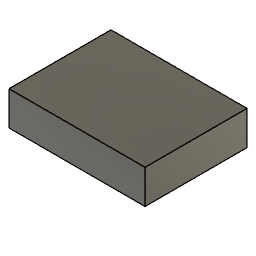
Cutting Block Tibia Shell (L&R) (Autodesk Fusion 360 design; units mm, degrees)
Autodesk Fusion 360 part; units mm, degrees
note: some values were not read from the file. Chosen so that the rebuilt part matches the saved one: which bodies a step acts on; which face or edge a step refers to. Set by a fixed rule: which sketch regions a step uses.
sketch "Sketch1" plane through (0, 0, 0) normal (0, 0, 1) x (1, 0, 0)
  line L0 (0, 64.6235) -> (0, -66.6531) construction
  line L1 (95.8471, 0) -> (-100, 0) construction
  circle A0 centre (18, 0) radius 20
  circle A1 centre (-18, 0) radius 20
  line L2 (40, 22) -> (-40, 22) construction
  line L3 (-40, 22) -> (-40, -22) construction
  line L4 (-40, -22) -> (40, -22) construction
  line L5 (40, -22) -> (40, 22) construction
  line L6 (40, 22) -> (-40, -22) construction
  line L7 (-40, 22) -> (40, -22) construction
  circle A2 centre (0, 80) radius 102
  line L8 (-18, 20) -> (18, 20)
  line L9 (-8.7733, 50.0836) -> (-8.7733, 13.6847)
  arc A3 (-8.7733, 13.6847) -> (8.7733, 13.6847) centre (0, 13.6847) ccw
  line L10 (8.7733, 13.6847) -> (8.7733, 50.0836)
  arc A4 (8.7733, 50.0836) -> (-8.7733, 50.0836) centre (0, 50.0836) ccw
  line L11 (0, 50.0836) -> (0, 13.6847) construction
  point P0 (0, 31.8841)
  dimension "d1" = 18
  dimension "d2" = 80
  dimension "d3" = 44
  dimension "d4" = 40
  constraint vertical L0
  constraint perpendicular L0 L1
  constraint coincident origin L0
  constraint coincident origin L1
  constraint coincident L1 A0.centre
  constraint coincident L1 A1.centre
  constraint equal A0 A1
  constraint horizontal L2
  constraint perpendicular L2 L3
  constraint parallel L2 L4
  constraint parallel L3 L5
  constraint coincident L6 origin
  constraint coincident L7 origin
  constraint symmetric L0 A0 A1
  constraint coincident L0 A2.centre
  constraint tangent A0 A2
  constraint tangent L4 A2
  constraint parallel L2 L8
  constraint tangent A1 L8
  constraint coincident A1 L8.start
  constraint coincident A0 L8.end
  constraint tangent L9 A3
  constraint tangent A3 L10
  constraint parallel L9 L10
  constraint tangent L10 A4
  constraint tangent L9 A4
  constraint coincident L0 A3.centre
  constraint perpendicular L8 L11
  constraint coincident L0 P0
  constraint midpoint L11 P0
  measures "d1" distance of L0 A0.centre
  measures "d2" distance of L2.start L2.end
  measures "d3" distance of L2.start L4.end
  measures "d4" diameter of A0
extrude "Extrude1" add sketch "Sketch1" along normal blind 5 contours A0 A1 A3 L10 | A0 L8 L10 | A0 A1 A2 | A0 A1 L9 A3 | A0 A1 A3 | A1 L8 L9 picked at (9.3284, -4.7386) picked at (-9.2755, -5.111) picked at (-0.6455, 1.124) makes body 1
fillet "Fillet2" radius 8 2 edges at (8.7733, 20, 2.5) (-8.7733, 20, 2.5) on bodies 1
extrude "Extrude3" add 1 faces at (0, -12.8446, 5) along direction (0, 0, 1) blind 5 separate body on bodies 1 makes body 2
shell "Shell2" thickness 2 removed faces 1 at (3.2154, -12.8497, 10) on bodies 2
sketch "Sketch4" plane through (0, 0, 0) normal (0, 0, -1) x (1, 0, 0)
  arc A0 (-16.6885, -20) -> (-8.729, -12.8035) centre (-16.6885, -12) ccw
  arc A1 (8.729, -12.8035) -> (-8.729, -12.8035) centre (0, -13.6847) ccw
  arc A2 (8.729, -12.8035) -> (16.6885, -20) centre (16.6885, -12) ccw
  line L0 (16.6885, -20) -> (18, -20)
  arc A3 (18, -20) -> (22.3902, 19.5122) centre (18, 0) ccw
  arc A4 (22.3902, 19.5122) -> (-22.3902, 19.5122) centre (0, -80) ccw
  arc A5 (-22.3902, 19.5122) -> (-18, -20) centre (-18, 0) ccw
  line L1 (-18, -20) -> (-16.6885, -20)
  circle A6 centre (0, 7) radius 3.5
  line L2 (0, 7) -> (14.0954, 1.8697) construction
  line L3 (-0.342, 6.0603) -> (13.7534, 0.93)
  arc A7 (13.7534, 0.93) -> (14.4374, 2.8094) centre (14.0954, 1.8697) ccw
  line L4 (14.4374, 2.8094) -> (0.342, 7.9397)
  arc A8 (0.342, 7.9397) -> (-0.342, 6.0603) centre (0, 7) ccw
  line L5 (0, 7) -> (14.0954, 1.8697) construction
  line L6 (0, -4.9114) -> (0, 22) construction
  line L7 (0, 7) -> (-14.0954, 1.8697) construction
  arc A9 (-14.4374, 2.8094) -> (-13.7534, 0.93) centre (-14.0954, 1.8697) ccw
  line L8 (0, 7) -> (-14.0954, 1.8697) construction
  arc A10 (0.342, 6.0603) -> (-0.342, 7.9397) centre (0, 7) ccw
  line L9 (-14.4374, 2.8094) -> (-0.342, 7.9397)
  line L10 (0.342, 6.0603) -> (-13.7534, 0.93)
  circle A11 centre (22, 10) radius 2.9
  circle A12 centre (22, -10) radius 2.9
  circle A13 centre (-22, 10) radius 2.9
  circle A14 centre (-22, -10) radius 2.9
  point P0 (0, 7)
  point P1 (-22.3902, 19.5122)
  point P2 (-18, 0)
  dimension "d18" = 7
  dimension "d19" = 7
  dimension "d20" = 2
  dimension "d21" = 70
  dimension "d22" = 15
  dimension "d32" = 5.8
  dimension "d33" = 22
  dimension "d34" = 20
  dimension "d35" = 10
  constraint vertical origin A6.centre
  constraint coincident P0 A6.centre
  constraint tangent L3 A7
  constraint tangent A7 L4
  constraint parallel L3 L4
  constraint tangent L4 A8
  constraint tangent L3 A8
  constraint coincident L2.end A7.centre
  constraint parallel L2 L5
  constraint midpoint A1 L6.start
  constraint midpoint A4 L6.end
  constraint symmetric P0 L6 A6.centre
  constraint symmetric L2.end L6 L7.end
  constraint symmetric L3.start L6 A10.start
  constraint symmetric L3.end L6 A9.end
  constraint symmetric A7.end L6 A9.start
  constraint symmetric L4.end L6 A10.end
  constraint symmetric A7 L6 A9
  constraint symmetric A8 L6 A10
  constraint equal A11 A12
  constraint vertical A11.centre A12.centre
  constraint symmetric A3.end L6 P1
  constraint symmetric A3.centre L6 P2
  constraint symmetric L6 A11 A13
  constraint symmetric L6 A12 A14
  measures "d18" diameter of A6
  measures "d19" distance of origin A6.centre
  measures "d20" distance of L3 L4
  measures "d21" angle of L2 L6
  measures "d22" distance of P0 L2.end
  measures "d32" diameter of A11
  measures "d33" distance of L6 A11.centre
  measures "d34" distance of A11.centre A12.centre
  measures "d35" vertical distance of origin A11.centre
extrude "Extrude4" add sketch "Sketch4" along normal blind 20 contours A6 L4 A8 A10 L9 | A6 L3 A8 L9 L10 | A6 A9 L9 L10 | A6 L3 A7 L4 | A6 L3 L4 A10 L10 | A6 L3 L10 bodies 1
sketch "Sketch5" plane through (0, 0, 0) normal (0, 1, 0) x (1, 0, 0)
  line L0 (0, -10) -> (0, 20) construction
  line L1 (-22.3902, -10) -> (22.3902, -10)
  line L2 (3.5, 20) -> (-3.5, 20)
  line L3 (0, 20) -> (16.4374, 20)
  line L4 (16.4374, 20) -> (16.4374, 0)
  line L5 (-22.3902, 0) -> (22.3902, 0)
  line L6 (14.4374, 0) -> (14.4374, 20)
  spline S0 degree 5 poles (0, 20) (0.3411, 19.8623) (1.0253, 19.654) (2.0582, 19.543) (3.4353, 19.7283) (5.0876, 20.1351) (6.592, 20.2718) (7.8837, 19.7528) (8.9451, 18.4166) (9.8035, 16.3217) (10.5137, 13.6618) (11.1462, 10.7153) (11.7741, 7.7829) (12.4628, 5.138) (13.2548, 2.959) (14.1714, 1.3345) (15.0111, 0.5059) (15.701, 0.1503) (16.1875, 0.0306) (16.4374, 0) knots 0 0 0 0 0 0 0.066667 0.133333 0.2 0.266667 0.333333 0.4 0.466667 0.533333 0.6 0.666667 0.733333 0.8 0.866667 0.933333 1 1 1 1 1 1
  line L7 (-3.7175, 21.5008) -> (3.7175, 18.4992)
  point P0 (7, 20)
  point P1 (12, 7)
  dimension "d25" = 2
  constraint vertical L0
  constraint coincident L0.start L1
  constraint coincident L0.end L2
  constraint coincident origin L0
  constraint perpendicular L0 L3
  constraint perpendicular L2 L4
  constraint coincident L4.end L5
  constraint midpoint L0.end L7
  measures "d25" distance of L4 L6
extrude "Extrude5" [suppressed]
mirror "Mirror1" [suppressed]
fillet "Fillet3" [suppressed]
extrude "Extrude6" add sketch "Sketch4" along normal blind 9 separate body contours A11 | A12 | A13 | A14 makes body 3 at (-19.1036, 10.1446, -6) makes body 4 at (24.8964, -9.8554, -6) makes body 5 at (-19.1036, -9.8554, -6) makes body 6 at (24.8964, 10.1446, -6)
chamfer "Chamfer1" distance 2.5 angle 45 4 edges at (-24.7037, 11.0487, -9) (19.2963, -8.9513, -9) (-24.7037, -8.9513, -9) (19.2963, 11.0487, -9) on bodies 3 4 5 6
combine "Combine1" operation add target body 1 tool bodies 6 4 2 3 5
move_face "OffsetFaces1" offset -1 1 faces at (0, -12.2976, 7) on bodies 1
sketch "Sketch6" plane through (0, 0, 10) normal (0, 0, 1) x (-1, 0, 0)
  arc A0 (10.7189, -12.6026) -> (16.6885, -18) centre (16.6885, -12) ccw
  arc A1 (10.7189, -12.6026) -> (-10.7189, -12.6026) centre (0, -13.6847) ccw
  arc A2 (-16.6885, -18) -> (-10.7189, -12.6026) centre (-16.6885, -12) ccw
  line L0 (-16.6885, -18) -> (-18, -18)
  arc A3 (-21.9512, 17.561) -> (-18, -18) centre (-18, 0) ccw
  arc A4 (21.9512, 17.561) -> (-21.9512, 17.561) centre (0, -80) ccw
  arc A5 (18, -18) -> (21.9512, 17.561) centre (18, 0) ccw
  line L1 (18, -18) -> (16.6885, -18)
  arc A6 (8.729, -12.8035) -> (16.6885, -20) centre (16.6885, -12) ccw
  line L2 (16.6885, -20) -> (18, -20)
  arc A7 (18, -20) -> (22.3902, 19.5122) centre (18, 0) ccw
  arc A8 (22.3902, 19.5122) -> (-22.3902, 19.5122) centre (0, -80) ccw
  arc A9 (-22.3902, 19.5122) -> (-18, -20) centre (-18, 0) ccw
  line L3 (-18, -20) -> (-16.6885, -20)
  arc A10 (-16.6885, -20) -> (-8.729, -12.8035) centre (-16.6885, -12) ccw
  arc A11 (8.729, -12.8035) -> (-8.729, -12.8035) centre (0, -13.6847) ccw
  line L4 (0, -4.9114) -> (0, 22)
  line L5 (1, -3.9114) -> (-1, -3.9114)
  line L6 (-1, -3.9114) -> (-1, 21)
  line L7 (-1, 21) -> (1, 21)
  line L8 (1, 21) -> (1, -3.9114)
  line L9 (2, -3.9114) -> (-2, -3.9114)
  line L10 (-2, -3.9114) -> (-2, 21)
  line L11 (-2, 21) -> (2, 21)
  line L12 (2, 21) -> (2, -3.9114)
  dimension "d40" = 2
  dimension "d41" = 1
  dimension "d42" = 1
  dimension "d44" = 2
  dimension "d45" = 1
  dimension "d46" = 1
  constraint midpoint A11 L4.start
  constraint midpoint A8 L4.end
  constraint horizontal L5
  constraint vertical L6
  constraint horizontal L7
  constraint vertical L8
  constraint horizontal L9
  constraint vertical L10
  constraint horizontal L11
  constraint vertical L12
  constraint collinear L5 L9
  constraint collinear L7 L11
  measures "d40" distance of L6 L8
  measures "d41" distance of L4.end L7
  measures "d42" distance of L4.start L5
  measures "d45" distance of L8 L12
  measures "d46" distance of L6 L10
extrude "Extrude7" add sketch "Sketch6" against normal up to surface (4 mm away) contours A1 A4 L4 L8 | A1 A4 L4 L6 bodies 1
extrude "Extrude8" add sketch "Sketch6" against normal blind 1 contours A1 A4 L8 L12 | A1 A4 L6 L10 bodies 1
chamfer "Chamfer3" distance 1 distance2 6.5 4 edges at (19.2963, -8.9513, -6.5) (19.2963, 11.0487, -6.5) (-24.7037, 11.0487, -6.5) (-24.7037, -8.9513, -6.5) measured on face at (21.1435, -7.8176, -7.0556) measured on face at (21.1435, 12.1824, -7.0556) measured on face at (-22.8565, 12.1824, -7.0556) measured on face at (-22.8565, -7.8176, -7.0556) on bodies 1
move_face "OffsetFaces2" offset -0.2 8 faces at (10.7896, -4.1371, -6.6667) (3.4994, -7.0641, -13.3333) (-10.7896, -4.1371, -6.6667) (-6.4577, -3.5854, -6.6667) (-1.0699, -3.6675, -13.3333) (6.4577, -3.5854, -13.3333) (14.3865, -0.913, -13.3333) (-13.9085, -0.8873, -13.3333) on bodies 1
sketch "Sketch7" plane through (0, 0, 0) normal (0, 0, -1) x (1, 0, 0)
  arc A0 (-16.6885, -20) -> (-8.729, -12.8035) centre (-16.6885, -12) ccw
  arc A1 (8.729, -12.8035) -> (-8.729, -12.8035) centre (0, -13.6847) ccw
  arc A2 (8.729, -12.8035) -> (16.6885, -20) centre (16.6885, -12) ccw
  line L0 (16.6885, -20) -> (18, -20)
  arc A3 (18, -20) -> (22.3902, 19.5122) centre (18, 0) ccw
  arc A4 (22.3902, 19.5122) -> (-22.3902, 19.5122) centre (0, -80) ccw
  arc A5 (-22.3902, 19.5122) -> (-18, -20) centre (-18, 0) ccw
  line L1 (-18, -20) -> (-16.6885, -20)
  line L2 (-14.369, 2.6215) -> (-3.2821, 6.6568)
  arc A6 (3.2821, 6.6568) -> (-3.2821, 6.6568) centre (0, 7) ccw
  line L3 (3.2821, 6.6568) -> (14.369, 2.6215)
  arc A7 (13.8218, 1.1179) -> (14.369, 2.6215) centre (14.0954, 1.8697) ccw
  line L4 (13.8218, 1.1179) -> (2.7349, 5.1532)
  arc A8 (-2.7349, 5.1532) -> (2.7349, 5.1532) centre (0, 7) ccw
  line L5 (-2.7349, 5.1532) -> (-13.8218, 1.1179)
  arc A9 (-14.369, 2.6215) -> (-13.8218, 1.1179) centre (-14.0954, 1.8697) ccw
  line L6 (80, 60) -> (-80, 60)
  line L7 (-80, 60) -> (-80, -60)
  line L8 (-80, -60) -> (80, -60)
  line L9 (80, -60) -> (80, 60)
  line L10 (80, 60) -> (-80, -60) construction
  line L11 (-80, 60) -> (80, -60) construction
  circle A10 centre (-22, 10) radius 2.9
  circle A11 centre (-22, -10) radius 2.9
  circle A12 centre (22, 10) radius 2.9
  circle A13 centre (22, -10) radius 2.9
  dimension "d56" = 120
  dimension "d57" = 160
  constraint horizontal L6
  constraint perpendicular L6 L7
  constraint parallel L6 L8
  constraint parallel L7 L9
  constraint coincident L10 origin
  constraint coincident L11 origin
  measures "d56" distance of L6.start L8.end
  measures "d57" distance of L6.start L6.end
extrude "Extrude9" add sketch "Sketch7" against normal blind 40 contours A0 A1 A2 L0 A3 A4 A5 L1 | L2 A6 L3 A7 L4 A8 L5 A9 | L6 L7 L8 L9 | A10 | A11 | A12 | A13 bodies 1
